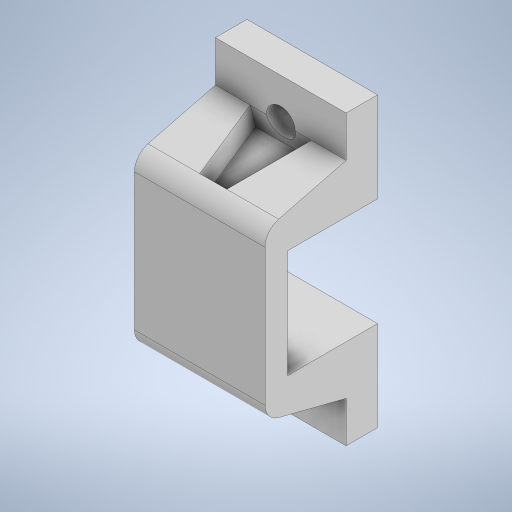
# Autodesk Inventor part: soporte_motor
Saved by Autodesk Inventor 2024 (Build 280153020, 153B)
## iProperties
Created: 2023-05-22
Part Number: soporte_motor
Material: Generic
Document SubType Name: Modeling
Designer: Diego
Density: 1 g/cm^3
Appearance: Default
Author: Diego
Autodesk Inventor part; units mm, degrees
ref_plane "YZ Plane" through (0, 0, 0) normal (1, 0, 0) x (0, 1, 0)
ref_plane "XZ Plane" through (0, 0, 0) normal (0, 1, 0) x (-1, 0, 0)
ref_plane "XY Plane" through (0, 0, 0) normal (0, 0, 1) x (1, 0, 0)
sketch "Sketch1" plane through (0, 0, 0) normal (1, 0, 0) x (0, 1, 0)
  line L0 (-6, -5) -> (0, -5) construction
  line L1 (6, -5) -> (6, 5)
  line L2 (6, 5) -> (-6, 5)
  line L3 (-6, 5) -> (-6, -5)
  line L4 (-6, -5) -> (6, 5) construction
  line L5 (6, -5) -> (-6, 5) construction
  line L6 (-7.5995, 7.5) -> (7.5995, 7.5)
  line L7 (9.1552, -7.5) -> (-9.1552, 7.5) construction
  line L8 (-9.1552, -7.5) -> (9.1552, 7.5) construction
  line L9 (9.1552, -7.5) -> (9, -7.5)
  line L10 (-9, -7.5) -> (-9.1552, -7.5)
  line L11 (-6, -5) -> (-16, -5)
  line L12 (-16, -5) -> (-16, -1.5)
  line L13 (-16, -1.5) -> (-11.44, -1.5)
  line L14 (-11.44, -1.5) -> (-9.538, 5.9921)
  line L15 (0, 0) -> (0, 13.1521) construction
  line L16 (9.1552, -7.5) -> (-9.1552, 7.5) construction
  line L17 (9, -7.5) -> (9.1552, -7.5)
  line L18 (6, -5) -> (16, -5)
  line L19 (16, -5) -> (16, -1.5)
  line L20 (16, -1.5) -> (11.44, -1.5)
  line L21 (11.44, -1.5) -> (9.538, 5.9921)
  arc A0 (-7.5995, 7.5) -> (-9.538, 5.9921) centre (-7.5995, 5.5) ccw
  arc A1 (9.538, 5.9921) -> (7.5995, 7.5) centre (7.5995, 5.5) ccw
  dimension "d0" = 12
  dimension "d1" = 10
  dimension "d2" = 2.5
  dimension "d3" = 10
  dimension "d4" = 3.5
  dimension "d5" = 4.56
  dimension "d6" = 2
  constraints: 44 end point, 7 point on line, 5 horizontal, 5 symmetric about line, 4 midpoint, 4 parallel, 4 point on circle, 4 tangent, 2 centre point, 2 vertical, 1 equal radius, 1 perpendicular
  measures "d0" distance of L2.end L1.end
  measures "d1" distance of L1.end L1.start
  measures "d2" distance between parallel lines of L6 L2
  measures "d3" distance of L0.start L11.end
  measures "d4" distance of L11.end L12.end
  measures "d5" distance of L12.end L13.end
  measures "d6" radius of A0
extrude "Extrusion1" add sketch "Sketch1" along normal blind 14.5
sketch "Sketch2" plane through (0, 9.538, 5.9921) normal (0, 0.9692541, 0.2460618) x (1, 0, 0)
  line L0 (0, 7.7298) -> (14.5, 7.7298) projected
  line L1 (7.25, 7.7298) -> (15.5846, 7.7298) construction
  line L2 (7.25, 7.7298) -> (7.25, 0) construction
  line L3 (7.25, 0) -> (8.75, 0)
  line L4 (0, 0) -> (14.5, 0) projected
  line L5 (7.25, 0) -> (5.75, 0)
  line L6 (7.25, 7.7298) -> (10.65, 7.7298)
  line L7 (7.25, 7.7298) -> (3.85, 7.7298)
  line L8 (3.85, 7.7298) -> (5.75, 0)
  line L9 (10.65, 7.7298) -> (8.75, 0)
  point P0 (0, 3.461)
  point P1 (10.65, 7.7298)
  dimension "d13" = 1.5
  dimension "d14" = 1.5
  dimension "d15" = 3.4
  dimension "d16" = 3.4
  constraints: 16 end point, 4 point on line, 1 horizontal, 1 midpoint
  measures "d13" distance of L2.end L3.end
  measures "d14" distance of L2.end L5.end
  measures "d15" distance of L1.start L6.end
  measures "d16" distance of L1.start L7.end
extrude "Extrusion2" cut sketch "Sketch2" against normal blind 2.5
sketch "Sketch3" plane through (0, 11.44, -1.5) normal (0, 0, 1) x (1, 0, 0)
  line L0 (0, 4.56) -> (14.5, 4.56) construction
  line L1 (14.5, 4.56) -> (7.25, 0) construction
  line L2 (3.85, 0) -> (10.65, 0) construction
  line L3 (0, 4.56) -> (7.25, 0) construction
  circle A0 centre (7.25, 0) radius 1.6
  point P0 (0, -11.44)
  dimension "d19" = 3.2
  constraints: 4 end point, 1 centre point, 1 coincident, 1 midpoint
  measures "d19" diameter of A0
extrude "Extrusion3" cut sketch "Sketch3" against normal blind 4
sketch "Sketch4" plane through (0, -11.44, -1.5) normal (0, -0.9692541, 0.2460618) x (1, 0, 0)
  line L0 (0, 0) -> (14.5, 0) projected
  line L1 (7.25, 0) -> (10.65, 0) construction
  line L2 (7.25, 0) -> (7.25, 7.6387) construction
  line L3 (7.25, 0) -> (3.85, 0) construction
  line L4 (7.25, 0) -> (10.65, 0)
  line L5 (7.25, 0) -> (3.85, 0)
  line L6 (7.25, 7.3642) -> (7.25, 7.7298) construction
  line L7 (0, 7.7298) -> (14.5, 7.7298) construction
  line L8 (7.25, 7.7298) -> (5.75, 7.7298)
  line L9 (7.25, 7.7298) -> (8.75, 7.7298)
  line L10 (3.85, 0) -> (5.75, 7.7298)
  line L11 (10.65, 0) -> (8.75, 7.7298)
  point P0 (0, 4.2688)
  dimension "d22" = 3.4
  dimension "d23" = 3.4
  dimension "d25" = 1.5
  dimension "d26" = 1.5
  constraints: 20 end point, 5 point on line, 2 collinear, 2 midpoint
  measures "d22" distance of L1.start L1.end
  measures "d23" distance of L1.start L3.end
  measures "d25" distance of L6.end L8.end
  measures "d26" distance of L6.end L9.end
extrude "Extrusion4" cut sketch "Sketch4" against normal blind 2.5
sketch "Sketch5" plane through (0, -16, -1.5) normal (0, 0, 1) x (1, 0, 0)
  line L0 (0, 4.56) -> (0, 0) construction
  line L1 (0, 0) -> (7.25, 4.56) construction
  line L2 (3.85, 4.56) -> (10.65, 4.56) construction
  line L3 (14.5, 4.56) -> (14.5, 0) construction
  line L4 (14.5, 0) -> (7.25, 4.56) construction
  circle A0 centre (7.25, 4.56) radius 1.6
  point P0 (0, 16)
  dimension "d29" = 3.2
  constraints: 4 end point, 1 centre point, 1 coincident, 1 midpoint
  measures "d29" diameter of A0
extrude "Extrusion5" cut sketch "Sketch5" against normal blind 4
body "Solid1"
